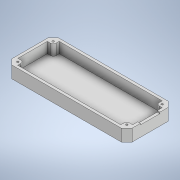
# Autodesk Inventor part: enclosed base
Saved by Autodesk Inventor 2022 (Build 260153000, 153)
## iProperties
Created: 2022-05-30
Part Number: enclosed base
Material: Generic
Document SubType Name: Modeling
Designer: Aakif
Density: 1 g/cm^3
Appearance: Default
Author: Aakif
Autodesk Inventor part; units mm, degrees
ref_plane "YZ Plane" through (0, 0, 0) normal (1, 0, 0) x (0, 1, 0)
ref_plane "XZ Plane" through (0, 0, 0) normal (0, 1, 0) x (-1, 0, 0)
ref_plane "XY Plane" through (0, 0, 0) normal (0, 0, 1) x (1, 0, 0)
sketch "Sketch1" plane through (0, 0, 0) normal (0, 1, 0) x (-1, 0, 0)
  line L0 (82, 35) -> (-82, 35)
  line L1 (-90, 27) -> (-90, -27)
  line L2 (-82, -35) -> (82, -35)
  line L3 (90, -27) -> (90, 27)
  line L4 (90, 35) -> (-90, -35) construction
  line L5 (-90, 35) -> (90, -35) construction
  line L6 (90, 27) -> (82, 35)
  line L7 (90, -27) -> (82, -35)
  line L8 (-82, 35) -> (-90, 27)
  line L9 (-82, -35) -> (-90, -27)
  point P0 (0, 0)
  dimension "d0" = 180
  dimension "d1" = 70
  dimension "d2" = 8
  dimension "d3" = 8
  dimension "d4" = 8
  dimension "d5" = 8
  dimension "d6" = 8
  dimension "d7" = 8
  dimension "d8" = 8
  dimension "d9" = 8
  constraints: 20 end point, 8 point on line, 2 midpoint, 2 parallel, 1 horizontal, 1 perpendicular
  measures "d0" distance of L5.end L4.end
  measures "d1" distance of L4.end L5.start
  measures "d2" distance of L3.end L4.start
  measures "d3" distance of L0.start L4.start
  measures "d4" distance of L3.start L5.end
  measures "d5" distance of L2.end L5.end
  measures "d6" distance of L0.end L5.start
  measures "d7" distance of L1.start L5.start
  measures "d8" distance of L2.start L4.end
  measures "d9" distance of L1.end L4.end
extrude "Extrusion1" add sketch "Sketch1" against normal blind 2
sketch "Sketch2" plane through (0, 0, 0) normal (0, 1, 0) x (1, 0, 0)
  line L0 (-82, -35) -> (82, -35)
  line L1 (90, -27) -> (90, 27)
  line L2 (82, 35) -> (-82, 35)
  line L3 (-90, 27) -> (-90, -27)
  line L4 (-90, -35) -> (90, 35) construction
  line L5 (90, -35) -> (-90, 35) construction
  line L6 (-90, -27) -> (-82, -35)
  line L7 (-90, 27) -> (-82, 35)
  line L8 (82, 35) -> (90, 27)
  line L9 (82, -35) -> (90, -27)
  line L10 (-86, -25.3431) -> (-80.3431, -31)
  line L11 (-80.3431, -31) -> (80.3431, -31)
  line L12 (80.3431, -31) -> (86, -25.3431)
  line L13 (86, -25.3431) -> (86, 25.3431)
  line L14 (86, 25.3431) -> (80.3431, 31)
  line L15 (80.3431, 31) -> (-80.3431, 31)
  line L16 (-80.3431, 31) -> (-86, 25.3431)
  line L17 (-86, 25.3431) -> (-86, -25.3431)
  line L18 (0, 0) -> (90, 0)
  line L19 (90, 0) -> (90, -14.5)
  line L20 (90, -14.5) -> (0, -14.5)
  line L21 (0, -14.5) -> (0, 0)
  line L22 (0, 0) -> (90, 0)
  line L23 (90, 0) -> (90, 14.5)
  line L24 (90, 14.5) -> (0, 14.5)
  line L25 (0, 14.5) -> (0, 0)
  line L26 (-90, 35) -> (-81.5147, 26.5147)
  circle A0 centre (-81.5147, 26.5147) radius 1.45
  circle A1 centre (-81.5147, 26.5147) radius 4.45
  line L27 (-90, 35) -> (-77.0647, 35)
  line L28 (-77.0647, 35) -> (-77.0647, 22.0647)
  line L29 (-77.0647, 22.0647) -> (-90, 22.0647)
  line L30 (-90, 22.0647) -> (-90, 35)
  circle A2 centre (-81.5147, -26.5147) radius 1.45
  circle A3 centre (-81.5147, -26.5147) radius 4.45
  line L31 (-90, -35) -> (-77.0647, -35)
  line L32 (-77.0647, -35) -> (-77.0647, -22.0647)
  line L33 (-77.0647, -22.0647) -> (-90, -22.0647)
  line L34 (-90, -22.0647) -> (-90, -35)
  circle A4 centre (81.5147, 26.5147) radius 1.45
  circle A5 centre (81.5147, 26.5147) radius 4.45
  line L35 (77.0647, 35) -> (77.0647, 22.0647)
  line L36 (77.0647, 22.0647) -> (90, 22.0647)
  line L37 (77.0647, -22.0647) -> (90, -22.0647)
  line L38 (77.0647, -35) -> (77.0647, -22.0647)
  circle A6 centre (81.5147, -26.5147) radius 4.45
  circle A7 centre (81.5147, -26.5147) radius 1.45
  line L39 (90, -35) -> (77.0647, -35)
  line L40 (90, -22.0647) -> (90, -35)
  point P0 (86, -14.5)
  point P1 (86, 14.5)
  point P2 (81.5147, 22.0647)
  point P3 (86, 22.0647)
  point P4 (77.0647, 31)
  point P5 (77.0647, 26.5147)
  point P6 (77.0647, -26.5147)
  point P7 (77.0647, -31)
  point P8 (86, -22.0647)
  point P9 (81.5147, -22.0647)
  point P10 (-77.0647, -26.5147)
  point P11 (-81.5147, -22.0647)
  point P12 (-86, -22.0647)
  point P13 (-77.0647, -31)
  point P14 (-86, 22.0647)
  point P15 (-81.5147, 22.0647)
  point P16 (-77.0647, 26.5147)
  point P17 (-77.0647, 31)
  dimension "d12" = 180
  dimension "d13" = 70
  dimension "d14" = 8
  dimension "d15" = 8
  dimension "d16" = 8
  dimension "d17" = 8
  dimension "d18" = 8
  dimension "d19" = 8
  dimension "d20" = 8
  dimension "d21" = 8
  dimension "d22" = 4
  dimension "d23" = 90
  dimension "d24" = 14.5
  dimension "d25" = 90
  dimension "d26" = 14.5
  dimension "d31" = 12
  dimension "d32" = 2.9
  dimension "d33" = 3
  constraints: 82 end point, 14 symmetric about line, 10 parallel, 8 centre point, 8 point on line, 5 perpendicular, 4 horizontal, 2 midpoint, 1 coincident, 13 other
  measures "d12" distance of L5.end L4.end
  measures "d13" distance of L4.end L5.start
  measures "d14" distance of L3.end L4.start
  measures "d15" distance of L0.start L4.start
  measures "d16" distance of L3.start L5.end
  measures "d17" distance of L2.end L5.end
  measures "d18" distance of L2.start L4.end
  measures "d19" distance of L1.end L4.end
  measures "d20" distance of L0.end L5.start
  measures "d21" distance of L1.start L5.start
  measures "d22" distance between parallel lines of L3 L17
  measures "d23" distance of L19.end L20.end
  measures "d24" distance of L18.end L19.end
  measures "d25" distance of L24.end L23.end
  measures "d26" distance of L23.end L22.end
  measures "d31" distance of L26.start L26.end
  measures "d32" diameter of A0
  measures "d33" radial gap between concentric circles of A0 A1
extrude "Extrusion2" add sketch "Sketch2" along normal blind 16 contours L6 L3 L33 L17 L10 A3 L11 L32 L0 | L32 L11 L38 L0 | L38 L11 L12 A6 L13 L37 L1 L9 L0 | L11 L10 A3 L32 | L3 L29 L17 L33 | L38 A6 L12 L11 | A3 L10 | L3 L7 L26 A1 L16 L17 L29 | L33 A3 L10 L17 | A6 L12 | A3 L10 | L17 L16 A1 L29 | L37 L13 L20 L1 | L12 A6 | L37 L13 L12 A6 | L7 L2 L28 L15 L16 A1 L26 | A1 L16 | A1 L16 L26 | L26 L16 A1 | A1 L16 L15 L28 | L2 L35 L15 L28 | L24 L13 L36 L1 | L2 L8 L1 L36 L13 L14 A5 L15 L35 | L15 L14 A5 L35 | A5 L14 | L36 A5 L14 L13 | A5 L14
extrude "Extrusion3" add sketch "Sketch2" along normal blind 14 contours L20 L13 L18 L1 | L18 L13 L24 L1
equation "\"d3\" = d2"
equation "\"d4\" = d2"
equation "\"d5\" = d4"
equation "\"d6\" = d2"
equation "\"d7\" = d6"
equation "\"d8\" = d2"
equation "\"d9\" = d8"
equation "\"d15\" = d14"
equation "\"d16\" = d14"
equation "\"d17\" = d16"
equation "\"d18\" = d14"
equation "\"d19\" = d18"
equation "\"d20\" = d14"
equation "\"d21\" = d20"
body "Solid1"
